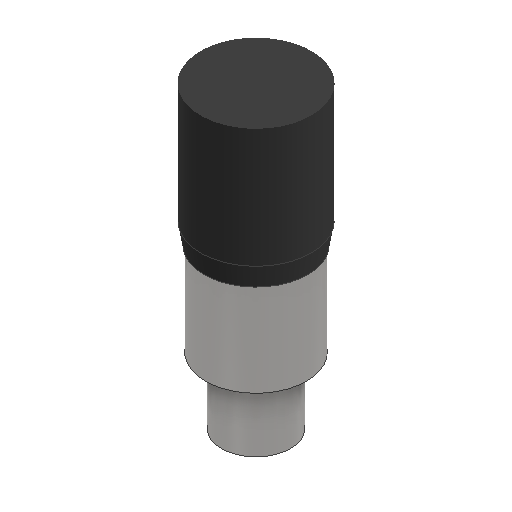
# Autodesk Inventor part: Rotary_handle
Saved by Autodesk Inventor 2026.2 (Build 302298000, 298)
## iProperties
Created: 2026-05-26
Part Number: Rotary_handle
Material: Generic
Document SubType Name: Modeling
Designer: zetsu
Density: 1 g/cm^3
Appearance: Default
Author: zetsu
Autodesk Inventor part; units mm, degrees
ref_plane "YZ Plane" through (0, 0, 0) normal (1, 0, 0) x (0, 1, 0)
ref_plane "XZ Plane" through (0, 0, 0) normal (0, 1, 0) x (-1, 0, 0)
ref_plane "XY Plane" through (0, 0, 0) normal (0, 0, 1) x (1, 0, 0)
sketch "スケッチ1" plane through (0, 0, 0) normal (0, 0, 1) x (1, 0, 0)
  line L0 (0, 0) -> (13, 0)
  line L1 (13, 0) -> (13, 25)
  line L2 (13, 25) -> (19, 25)
  line L3 (19, 25) -> (19, 60)
  line L4 (20.8, 67.7) -> (20.8, 112.7)
  line L5 (20.8, 112.7) -> (0, 112.7)
  line L6 (0, 112.7) -> (0, 0)
  line L7 (20.8, 67.7) -> (19.5, 60)
  line L8 (19.5, 60) -> (19, 60)
  dimension "d0" = 13
  dimension "d1" = 25
  dimension "d2" = 6
  dimension "d3" = 35
  dimension "d4" = 45
  dimension "d5" = 7.7
  dimension "d6" = 20.8
  dimension "d8" = 0.5
  constraints: 18 end point, 5 perpendicular, 2 horizontal, 1 parallel
  measures "d0" distance of L0.start L0.end
  measures "d1" distance of L0.end L1.end
  measures "d2" distance of L1.end L2.end
  measures "d3" distance of L2.end L3.end
  measures "d4" distance of L4.start L4.end
  measures "d5" vertical distance of L3.end L4.start
  measures "d6" distance of L4.end L5.end
  measures "d8" distance of L7.end L3.end
revolve "回転1" add sketch "スケッチ1" angle 360 about axis through (0, 112.7, 0) along (0, -1, 0)
